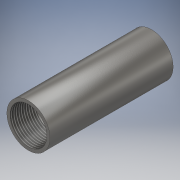
# Autodesk Inventor part: tube_reservoir
Saved by Autodesk Inventor 2019 (Build 230136000, 136)
## iProperties
Created: 2019-03-25
Part Number: tube_reservoir
Material: Acier, galvanisé
Document SubType Name: Modeling
Designer: theor
Density: 7.85 g/cm^3
Appearance: Galvanisé
Mass: 200.375 g
Surface Area: 209.309 cm^2
Volume: 25.5254 cm^3
Author: theor
Autodesk Inventor part; units mm, degrees
ref_plane "YZ Plane" through (0, 0, 0) normal (1, 0, 0) x (0, 1, 0)
ref_plane "XZ Plane" through (0, 0, 0) normal (0, 1, 0) x (-1, 0, 0)
ref_plane "XY Plane" through (0, 0, 0) normal (0, 0, 1) x (1, 0, 0)
sketch "Esquisse1" plane through (0, 0, 0) normal (0, 0, 1) x (1, 0, 0)
  circle A0 centre (0, 0) radius 15
  circle A1 centre (0, 0) radius 17.5
  dimension "d0" = 2.5
  dimension "d1" = 35
  dimension "d6" = 30
  constraints: 2 centre point, 2 coincident
  measures "d0" radial gap between concentric circles of A1 A0
  measures "d1" diameter of A1
  measures "d6" diameter of A0
extrude "Extrusion1" add sketch "Esquisse1" along normal blind 100
thread "Filetage1" size "M30x2" class "6H" standard "ISO Metric profile" length 20
